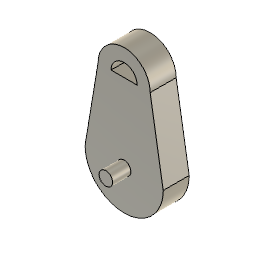
doorHinge.f3d (Autodesk Fusion 360 design; units mm, degrees)
Autodesk Fusion 360 part; units mm, degrees
sketch "Sketch1" plane through (0, 0, 0) normal (0, 1, 0) x (1, 0, 0)
  circle A0 centre (0, 0) radius 2.6
  circle A1 centre (0, 0) radius 15 construction
  arc A2 (15, 0) -> (-15, 0) centre (0, 0) ccw
  line L0 (-15, 0) -> (-10, -30)
  line L1 (15, 0) -> (10, -30)
  arc A3 (-10, -30) -> (10, -30) centre (0, -30) ccw
  line L2 (-5, -30) -> (5, -30)
  arc A4 (-5, -30) -> (5, -30) centre (0, -30) ccw
  dimension "d1" = 5.2
  dimension "d2" = 30
  constraint coincident A0.centre A1.centre
  constraint concentric A0 A1
  constraint coincident A1 A2.start
  constraint coincident A1 A2.end
  constraint horizontal L2
  constraint coincident A3.centre A4.centre
  measures "d1" diameter of A0
  measures "d2" diameter of A1
extrude "Extrude1" add sketch "Sketch1" along normal blind 10 contours A0 | A2 L0 L1 A3
extrude "Extrude2" add sketch "Sketch1" against normal blind 7 contours A0
